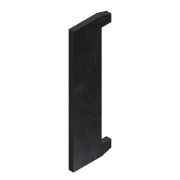
# Autodesk Inventor part: Left Side
Saved by Autodesk Inventor 2016 (Build 200138000, 138)
## iProperties
Created: 2015-05-19
Part Number: Left Side
Material: Steel
Document SubType Name: Modeling
Designer: Andy
Density: 7.85 g/cm^3
Appearance: Plate
Mass: 1194.77 g
Surface Area: 372.976 cm^2
Volume: 152.2 cm^3
Author: Andy
Autodesk Inventor part; units mm, degrees
ref_plane "YZ Plane" through (0, 0, 0) normal (1, 0, 0) x (0, 1, 0)
ref_plane "XZ Plane" through (0, 0, 0) normal (0, 1, 0) x (-1, 0, 0)
ref_plane "XY Plane" through (0, 0, 0) normal (0, 0, 1) x (1, 0, 0)
sketch "Sketch1" plane through (0, 0, 0) normal (1, 0, 0) x (0, 1, 0)
  line L0 (0, 0) -> (58, 0)
  line L1 (58, -250) -> (0, -250)
  line L2 (78, -6) -> (78, -21)
  line L3 (78, -21) -> (58, -21)
  line L4 (58, -21) -> (58, -125)
  line L5 (78, -21) -> (78, -6)
  line L6 (78, -21) -> (78, -6)
  line L7 (58, -229) -> (58, -125)
  line L8 (78, -229) -> (58, -229)
  line L9 (78, -244) -> (58, -250)
  line L10 (78, -244) -> (78, -229)
  line L11 (0, 0) -> (0, -62)
  line L12 (78, -6) -> (78, -21)
  line L13 (78, -229) -> (78, -244)
  line L14 (0, -250) -> (0, -75)
  line L15 (0, -62) -> (0, 0)
  line L16 (58, 0) -> (0, 0)
  line L17 (0, 0) -> (0, -62)
  line L18 (0, -75) -> (0, -250)
  line L19 (0, -250) -> (58, -250)
  line L20 (58, 0) -> (0, 0)
  line L21 (0, -62) -> (0, -75)
  line L22 (78, -6) -> (58, 0)
  dimension "d0" = 62
  dimension "d4" = 15
  dimension "d5" = 15
  dimension "d6" = 208
  constraints: 46 end point, 6 collinear, 5 parallel, 3 perpendicular, 2 horizontal, 1 vertical
  measures "d0" distance of L0.start L11.end
  measures "d4" distance of L10.start L8.start
  measures "d5" distance of L2.start L2.end
  measures "d6" distance between parallel lines of L3 L8
extrude "Extrusion1" add sketch "Sketch1" along normal blind 10
body "Solid1"
